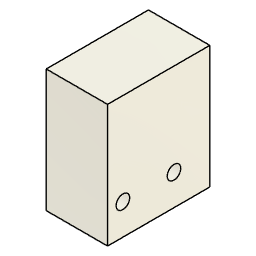
LoadcellBase (Autodesk Fusion 360 design; units mm, degrees)
Autodesk Fusion 360 part; units mm, degrees
sketch "Sketch1" plane through (0, 0, 0) normal (1, 0, 0) x (0, 1, 0)
  line L0 (0, 0) -> (30, 0)
  line L1 (30, 0) -> (30, 36)
  line L2 (30, 36) -> (0, 36)
  line L3 (0, 36) -> (0, 0)
  dimension "d1_1" = 30
  dimension "d2_1" = 36
  constraint horizontal L0
  constraint vertical L1
  constraint horizontal L2
  constraint vertical L3
  constraint coincident L0.start L3.end
  measures "d1_1" distance of L0.start L0.end
  measures "d2_1" distance of L0.start L2.end
extrude "Extrude1" add sketch "Sketch1" along normal blind 18
sketch "Sketch2" plane through (18, 0, 0) normal (1, 0, 0) x (0, 1, 0)
  line L0 (0, 36) -> (0, 0)
  line L1 (0, 0) -> (30, 0)
  line L2 (30, 0) -> (30, 36)
  line L3 (30, 36) -> (0, 36)
  line L4 (4.5, 0) -> (4.5, 9) construction
  line L5 (4.5, 9) -> (0, 9) construction
  circle A0 centre (4.5, 9) radius 2
  line L6 (4.5, 9) -> (19.5, 9) construction
  circle A1 centre (19.5, 9) radius 2
  dimension "d5_1" = 9
  dimension "d7_1" = 4.5
  dimension "d8_1" = 4
  dimension "d9" = 15
  dimension "d10" = 4
  constraint coincident L1 L4.start
  constraint perpendicular L1 L4
  constraint coincident L0 L5.end
  constraint perpendicular L0 L5
  constraint coincident L4.end L5.start
  constraint perpendicular L4 L6
  constraint coincident L6.end A1.centre
  measures "d5_1" distance of L4.start L4.end
  measures "d7_1" distance of L4.end L5.end
  measures "d8_1" diameter of A0
  measures "d9" distance of L4.end L6.end
  measures "d10" diameter of A1
extrude "Extrude2" cut sketch "Sketch2" against normal blind 18 contours A0 | A1
